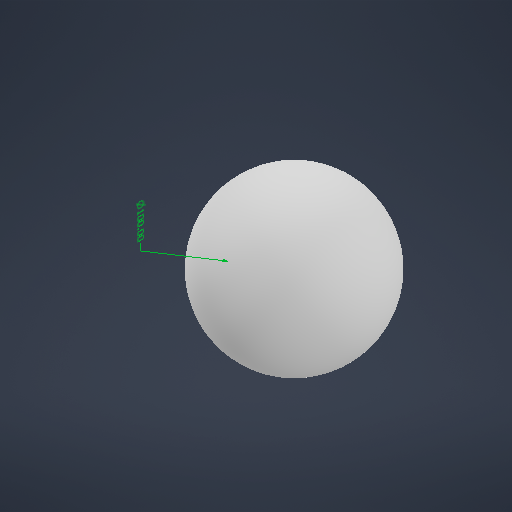
# Autodesk Inventor part: Objective_10mm_Ball_Manual
Saved by Autodesk Inventor 2026.1 (Build 301233020, 233B)
## iProperties
Created: 2025-10-17
Part Number: Objective_10mm_Ball_Manual
Material: Generic
Document SubType Name: Modeling
Designer: Asus
Density: 1 g/cm^3
Appearance: Default
Author: Asus
Autodesk Inventor part; units mm, degrees
ref_plane "YZ Plane" through (0, 0, 0) normal (1, 0, 0) x (0, 1, 0)
ref_plane "XZ Plane" through (0, 0, 0) normal (0, 1, 0) x (-1, 0, 0)
ref_plane "XY Plane" through (0, 0, 0) normal (0, 0, 1) x (1, 0, 0)
sketch "Sketch1" plane through (0, 0, 0) normal (0, 1, 0) x (-1, 0, 0)
  circle A0 centre (0, 0) radius 50
  line L0 (0, 50) -> (0, -50)
  dimension "d0" = 100
  constraints: 2 end point, 2 point on circle, 1 centre point, 1 coincident, 1 vertical
  measures "d0" diameter of A0
revolve "Revolution1" add sketch "Sketch1" angle 360 about axis through (0, 0, 50) along (0, 0, -1) picked at (11.7851, 11.7851) contours A0 L0
body "Solid1"
